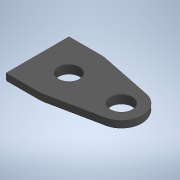
# Autodesk Inventor part: block_02
Saved by Autodesk Inventor 2020 (Build 240168000, 168)
## iProperties
Created: 2022-07-31
Part Number: block_02
Material: Типовые
Document SubType Name: Modeling
Designer: akapu
Density: 1 g/cm^3
Appearance: По умолчанию
Author: akapu
Autodesk Inventor part; units mm, degrees
ref_plane "YZ Plane" through (0, 0, 0) normal (1, 0, 0) x (0, 1, 0)
ref_plane "XZ Plane" through (0, 0, 0) normal (0, 1, 0) x (-1, 0, 0)
ref_plane "XY Plane" through (0, 0, 0) normal (0, 0, 1) x (1, 0, 0)
sketch "Эскиз1" plane through (0, 0, 0) normal (0, 1, 0) x (-1, 0, 0)
  circle A0 centre (0, 0) radius 2.5
  circle A1 centre (0, 0) radius 7.5
  line L0 (0, 7.5) -> (7.5, 7.5)
  line L1 (7.5, 7.5) -> (7.5, -7.5)
  line L2 (7.5, -7.5) -> (0, -7.5)
  line L3 (0, -7.5) -> (0, 7.5)
  line L4 (-7.5, 0) -> (-12.5, 0)
  circle A2 centre (-12.5, 0) radius 2.6
  circle A3 centre (-12.5, 0) radius 5
  line L5 (-1.5661, 7.3347) -> (-13.4999, 4.899)
  line L6 (-13.5, -4.899) -> (-1.5, -7.3485)
  dimension "d0" = 5
  dimension "d1" = 15
  dimension "d2" = 5
  dimension "d3" = 5.2
  constraints: 14 end point, 7 point on circle, 4 centre point, 4 coincident, 3 tangent, 2 horizontal, 2 parallel, 1 perpendicular
  measures "d0" diameter of A0
  measures "d1" diameter of A1
  measures "d2" distance of L4.start L4.end
  measures "d3" diameter of A2
extrude "Выдавливание1" add sketch "Эскиз1" along normal blind 2 contours A0 L3 A1 | A0 L3 A1 | L0 L1 A1 | A1 L1 L2 | A1 A3 L5 | L6 A3 A1 | A3
fillet "Сопряжение1" radius 0.7 8 edges at (0.7874, 0, 7.4586) (-3.75, 0, 7.5) (-7.5, 0, 0) (0.7538, 0, -7.462) (7.5, 0, -6.1237) (17.5, 0, 0.0001) (7.533, 0, 6.1168) (-3.75, 0, -7.5)
